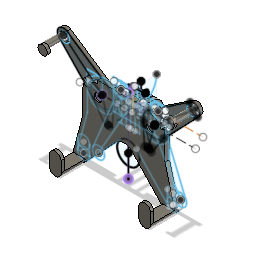
phone_holder (Autodesk Fusion 360 design; units mm, degrees)
Autodesk Fusion 360 part; units mm, degrees
sketch "Sketch1" plane through (0, 0, 0) normal (0, 0, 1) x (1, 0, 0)
  line L0 (-0.0193, 69.85) -> (19.0307, 69.85)
  line L1 (19.0307, 69.85) -> (19.0307, 50.8)
  line L2 (19.0307, 50.8) -> (-0.0193, 50.8)
  line L3 (-0.0193, 50.8) -> (-0.0193, 69.85)
  line L4 (3.7907, 69.85) -> (3.7907, 50.8)
  line L5 (7.6007, 69.85) -> (7.6007, 50.8)
  line L6 (11.4107, 69.85) -> (11.4107, 50.8)
  line L7 (15.2207, 69.85) -> (15.2207, 50.8)
  line L8 (-0.0193, 50.8) -> (-25.4193, 6.8059)
  line L9 (-0.0193, 50.8) -> (-41.2667, 50.8) construction
  line L10 (19.0307, 50.8) -> (44.4307, 6.8059)
  line L11 (19.0307, 50.8) -> (57.15, 50.8) construction
  circle A0 centre (-25.4193, 6.8059) radius 2.54
  circle A1 centre (44.4307, 6.8059) radius 2.54
  circle A2 centre (-25.4193, 6.8059) radius 5.08
  circle A3 centre (44.4307, 6.8059) radius 5.08
  line L12 (-12.7193, 68.9588) -> (31.7307, 68.9588)
  line L13 (31.7307, 68.9588) -> (31.7307, 43.5588)
  line L14 (31.7307, 43.5588) -> (-12.7193, 43.5588)
  line L15 (-12.7193, 43.5588) -> (-12.7193, 68.9588)
  line L16 (-12.7193, 50.8) -> (-30.1136, 8.7476)
  line L17 (31.7307, 50.8) -> (49.1249, 8.7476)
  circle A4 centre (-6.3693, 62.6088) radius 1.5875
  circle A5 centre (25.3807, 62.6088) radius 1.5875
  line L18 (-6.3693, 62.6088) -> (31.75, 62.6088) construction
  line L19 (25.3807, 62.6088) -> (63.5, 62.6088) construction
  circle A6 centre (-6.3693, 62.6088) radius 6.35
  circle A7 centre (25.3807, 62.6088) radius 6.35
  circle A8 centre (25.3807, 62.6088) radius 5.715
  circle A9 centre (-6.3693, 62.6088) radius 5.715
  line L20 (-6.3693, 68.9588) -> (-6.3693, 62.6088)
  line L21 (25.3807, 68.9588) -> (25.3807, 62.6088)
  line L22 (25.3807, 62.6088) -> (31.2629, 66.005)
  line L23 (25.3807, 62.6088) -> (31.75, 62.6088) construction
  line L24 (-6.3693, 62.6088) -> (-12.2226, 65.9882)
  line L25 (-6.3693, 62.6088) -> (-2.5108, 62.6088) construction
  circle A10 centre (25.3807, 62.6088) radius 1.4605
  circle A11 centre (-6.3693, 62.6088) radius 1.4605
  line L26 (29.6822, 66.3715) -> (31.731, 66.3715) construction
  line L27 (25.3807, 62.6088) -> (38.0807, 62.6088) construction
  line L28 (-6.3693, 62.6088) -> (12.6807, 62.6088) construction
  point P0 (-6.3693, 62.6088)
  point P1 (25.3807, 62.6088)
  dimension "d1" = 19.05
  dimension "d2" = 3.81
  dimension "d3" = 3.81
  dimension "d4" = 3.81
  dimension "d5" = 3.81
  dimension "d6" = 19.05
  dimension "d7" = 50.8
  dimension "d10" = 120
  dimension "d11" = 50.8
  dimension "d12" = 60
  dimension "d13" = 50.8
  dimension "d14" = 5.08
  dimension "d15" = 5.08
  dimension "d16" = 10.16
  dimension "d17" = 10.16
  dimension "d19" = 44.45
  dimension "d21" = 12.7
  dimension "d34" = 6.35
  dimension "d35" = 6.35
  dimension "d36" = 3.175
  dimension "d37" = 3.175
  dimension "d42" = 12.7
  dimension "d43" = 12.7
  dimension "d44" = 6.35
  dimension "d45" = 11.43
  dimension "d46" = 11.43
  dimension "d47" = 30
  dimension "d48" = 150
  dimension "d53" = 2.921
  dimension "d60" = 2.921
  constraint horizontal L0
  constraint vertical L1
  constraint horizontal L2
  constraint vertical L3
  constraint coincident L0 L4.start
  constraint coincident L2 L4.end
  constraint perpendicular L2 L4
  constraint coincident L0 L5.start
  constraint coincident L2 L5.end
  constraint perpendicular L2 L5
  constraint coincident L0 L6.start
  constraint coincident L2 L6.end
  constraint perpendicular L2 L6
  constraint coincident L0 L7.start
  constraint coincident L2 L7.end
  constraint perpendicular L2 L7
  constraint horizontal L9
  constraint horizontal L11
  constraint coincident L8.end A0.centre
  constraint coincident L10.end A1.centre
  constraint concentric A0 A2
  constraint concentric A1 A3
  constraint horizontal L12
  constraint vertical L13
  constraint horizontal L14
  constraint vertical L15
  constraint coincident L9 L16.start
  constraint coincident L15 L16.start
  constraint coincident A2 L16.end
  constraint tangent A2 L16
  constraint coincident L11 L17.start
  constraint coincident L13 L17.start
  constraint coincident A3 L17.end
  constraint tangent A3 L17
  constraint horizontal P0 P1
  constraint coincident P0 A4.centre
  constraint coincident P1 A5.centre
  constraint horizontal L18
  constraint horizontal L19
  constraint concentric A4 A6
  constraint concentric A5 A7
  constraint coincident L12 L20.start
  constraint coincident A6 L20.start
  constraint coincident L12 L21.start
  constraint coincident A7 L21.start
  constraint perpendicular L18 L21
  constraint horizontal L23
  constraint horizontal L25
  constraint concentric A7 A10
  constraint horizontal L26
  constraint coincident A8 L26.start
  constraint horizontal L27
  constraint horizontal L28
  measures "d1" distance of L0.start L2.end
  measures "d2" distance of L0.start L4
  measures "d3" distance of L4 L5
  measures "d4" distance of L5 L6
  measures "d5" distance of L6 L7
  measures "d6" distance of L1 L3
  measures "d7" distance of origin L2
  measures "d10" angle of L8 L9
  measures "d11" distance of L2.end L8.end
  measures "d12" angle of L10 L11
  measures "d13" distance of L1.end L10.end
  measures "d14" diameter of A0
  measures "d15" diameter of A1
  measures "d16" diameter of A2
  measures "d17" diameter of A3
  measures "d19" distance of L12.start L12.end
  measures "d21" horizontal distance of L0.start L12.start
  measures "d34" distance of L12 P0
  measures "d35" horizontal distance of L12.start P0
  measures "d36" diameter of A4
  measures "d37" diameter of A5
  measures "d42" diameter of A6
  measures "d43" diameter of A7
  measures "d44" distance of L13 P1
  measures "d45" diameter of A8
  measures "d46" diameter of A9
  measures "d47" angle of L22 L23
  measures "d48" angle of L24 L25
  measures "d53" diameter of A10
  measures "d60" diameter of A11
sketch "Sketch2" plane through (3.7907, 0, 0) normal (-1, 0, 0) x (0, 0, 1)
  line L0 (0, 68.9588) -> (-20.32, 68.9588)
  line L1 (-20.32, 68.9588) -> (-20.32, 50.8)
  line L2 (-20.32, 50.8) -> (0, 50.8)
  circle A0 centre (-10.795, 59.8794) radius 2.54
  arc A1 (-20.3135, 68.9588) -> (-2.7389, 50.8) centre (-1.6346, 69.4527) ccw
  line L3 (0, 50.8) -> (0, 68.9588)
  point P0 (-10.795, 59.8794)
  point P1 (0, 69.85)
  dimension "d125" = 9.525
  dimension "d126" = 5.08
  dimension "d127" = 9.0794
  constraint coincident P0 A0.centre
  constraint tangent L1 A1
  constraint coincident L2 A1.end
  constraint coincident L0 A1.start
  measures "d125" horizontal distance of L0.end P0
  measures "d126" diameter of A0
  measures "d127" distance of L0 P0
sketch "Sketch3" plane through (0, 0, 0) normal (0, 0, 1) x (1, 0, 0)
  line L0 (0, 0) -> (0, 63.5)
  line L1 (-9.525, 63.5092) -> (0, 63.5)
  circle A0 centre (0, 19.05) radius 9.525
  circle A1 centre (-38.0999, 0.0651) radius 2.54
  circle A2 centre (-38.0999, 0.0651) radius 5.08
  line L2 (-34.4118, -3.4284) -> (-6.9152, 25.6002)
  line L3 (-9.525, 63.5092) -> (-34.925, 63.5092)
  line L4 (-34.925, 63.5092) -> (-34.925, 31.7592)
  line L5 (-34.925, 31.7592) -> (-43.0092, 1.3711)
  line L6 (-9.525, 63.5092) -> (-9.525, 38.1092)
  line L7 (-9.525, 38.1092) -> (0, 38.1092)
  line L8 (-9.525, 57.1592) -> (0, 57.1592)
  line L9 (-5.715, 57.1592) -> (-5.715, 38.1092)
  line L10 (-1.905, 57.1592) -> (-1.905, 38.1092)
  circle A3 centre (-22.225, 50.8092) radius 12.7
  circle A4 centre (-22.225, 50.8092) radius 10.16
  line L11 (-22.225, 50.8092) -> (-22.225, 63.5092)
  line L12 (-22.225, 50.8092) -> (-34.1591, 55.1529)
  line L13 (-22.225, 50.8092) -> (-9.525, 50.8092) construction
  circle A5 centre (-22.225, 50.8092) radius 1.4605
  line L14 (9.525, 63.5092) -> (9.525, 38.1092)
  line L15 (34.925, 31.7592) -> (43.0092, 1.3711)
  line L16 (9.525, 63.5092) -> (34.925, 63.5092)
  circle A6 centre (38.0999, 0.0651) radius 2.54
  line L17 (9.525, 57.1592) -> (0, 57.1592)
  line L18 (34.4118, -3.4284) -> (6.9152, 25.6002)
  line L19 (5.715, 57.1592) -> (5.715, 38.1092)
  line L20 (22.225, 50.8092) -> (22.225, 63.5092)
  line L21 (1.905, 57.1592) -> (1.905, 38.1092)
  line L22 (22.225, 50.8092) -> (34.1591, 55.1529)
  circle A7 centre (22.225, 50.8092) radius 12.7
  circle A8 centre (0, 19.05) radius 9.525
  line L23 (9.525, 63.5092) -> (0, 63.5)
  circle A9 centre (22.225, 50.8092) radius 1.4605
  line L24 (34.925, 63.5092) -> (34.925, 31.7592)
  circle A10 centre (38.0999, 0.0651) radius 5.08
  line L25 (9.525, 38.1092) -> (0, 38.1092)
  circle A11 centre (22.225, 50.8092) radius 10.16
  line L26 (22.225, 50.8092) -> (9.525, 50.8092) construction
  circle A12 centre (-38.0999, 8.359) radius 5.08
  line L27 (-43.1364, 9.0231) -> (-43.1799, 0.0898)
  line L28 (-33.0635, 9.0231) -> (-33.02, 0.0898)
  circle A13 centre (38.0999, 8.359) radius 5.08
  line L29 (33.0635, 9.0231) -> (33.02, 0.0898)
  line L30 (43.1364, 9.0231) -> (43.1799, 0.0898)
  line L31 (43.1799, 0.0898) -> (33.02, 0.0898)
  line L32 (-33.02, 0.0898) -> (-43.1799, 0.0898)
  circle A14 centre (-22.225, 50.8092) radius 3.175
  circle A15 centre (22.225, 50.8092) radius 3.175
  point P0 (-38.0999, 0.0651)
  point P1 (13.8708, 60.4993)
  point P2 (-22.225, 50.8092)
  point P3 (22.225, 50.8092)
  point P4 (38.0999, 0.0651)
  dimension "d130" = 63.5
  dimension "d131" = 38.1
  dimension "d134" = 19.05
  dimension "d135" = 19.05
  dimension "d136" = 5.08
  dimension "d137" = 10.16
  dimension "d138" = 25.4
  dimension "d139" = 31.75
  dimension "d140" = 25.4
  dimension "d141" = 6.35
  dimension "d145" = 12.7
  dimension "d146" = 12.7
  dimension "d148" = 3.81
  dimension "d149" = 3.81
  dimension "d150" = 25.4
  dimension "d151" = 20.32
  dimension "d152" = 160
  dimension "d153" = 2.921
  dimension "d159" = 10.16
  dimension "d166" = 6.35
  constraint coincident L0.start origin
  constraint vertical L0
  constraint coincident L0 A0.centre
  constraint coincident P0 A1.centre
  constraint coincident A2 L2.start
  constraint coincident A0 L2.end
  constraint tangent A0 L2
  constraint tangent A2 L2
  constraint perpendicular L3 L4
  constraint coincident A2 L5.end
  constraint tangent A2 L5
  constraint perpendicular L3 L6
  constraint coincident L0 L7.end
  constraint perpendicular L0 L7
  constraint coincident L6 L8.start
  constraint coincident L0 L8.end
  constraint perpendicular L0 L8
  constraint coincident L8 L9.start
  constraint coincident L7 L9.end
  constraint perpendicular L7 L9
  constraint coincident L8 L10.start
  constraint coincident L7 L10.end
  constraint perpendicular L7 L10
  constraint coincident P2 A3.centre
  constraint midpoint L3 L11.end
  constraint horizontal L13
  constraint concentric A3 A5
  constraint symmetric L1.end L0 L23.end
  constraint symmetric L0 P0 P4
  constraint symmetric L0 L1.start L14.start
  constraint symmetric L0 A0 A8
  constraint symmetric L0 A1 A6
  constraint symmetric L0 A2 A10
  constraint symmetric L0 L2.start L18.start
  constraint symmetric L0 L2.end L18.end
  constraint symmetric L0 L3.end L16.end
  constraint symmetric L0 L4.end L15.start
  constraint symmetric L0 L5.end L15.end
  constraint symmetric L0 L6.end L14.end
  constraint symmetric L0 L7.end L25.end
  constraint symmetric L0 L8.start L17.start
  constraint symmetric L0 L8.end L17.end
  constraint symmetric L0 P2 P3
  constraint symmetric L0 L9.start L19.start
  constraint symmetric L0 L9.end L19.end
  constraint symmetric L0 L10.start L21.start
  constraint symmetric L0 L10.end L21.end
  constraint symmetric L0 A3 A7
  constraint symmetric L0 A4 A11
  constraint symmetric L0 L11.end L20.end
  constraint symmetric L0 L12.end L22.end
  constraint symmetric L0 L13.end L26.end
  constraint symmetric L0 A5 A9
  constraint coincident A12 L27.start
  constraint coincident A2 L27.end
  constraint tangent A2 L27
  constraint coincident A12 L28.start
  constraint coincident A2 L28.end
  constraint tangent A2 L28
  constraint symmetric L0 A12 A13
  constraint symmetric L0 L27.start L30.start
  constraint symmetric L0 L27.end L30.end
  constraint symmetric L0 L28.start L29.start
  constraint symmetric L0 L28.end L29.end
  constraint horizontal L31
  constraint symmetric L0 A14 A15
  measures "d130" distance of L0.start L0.end
  measures "d131" distance of L0.start P0
  measures "d134" diameter of A0
  measures "d135" distance of L0.start A0.centre
  measures "d136" diameter of A1
  measures "d137" diameter of A2
  measures "d138" distance of L1.start L3.end
  measures "d139" distance of L3.end L4.end
  measures "d140" distance of L1.start L6.end
  measures "d141" distance of L1.start L8.start
  measures "d145" distance of L4 P2
  measures "d146" distance of L3 P2
  measures "d148" distance of L6 L9
  measures "d149" distance of L9 L10
  measures "d150" diameter of A3
  measures "d151" diameter of A4
  measures "d152" angle of L12 L13
  measures "d153" diameter of A5
  measures "d159" diameter of A12
  measures "d166" diameter of A14
extrude "Extrude27" add sketch "Sketch3" along normal blind 3.81 contours L0 L7 L8 L10 | L0 A0 L14 L15 L18 A7 A8 L24 A10 L25 A13 L29 | L0 A0 A2 L2 L4 L5 L6 L7 A3 A8 A12 L28 | L0 L17 L21 L25 | L0 L1 L6 L8 | L0 L14 L17 L23 | L7 L8 L9 L10 | L17 L19 L21 L25 | L6 L7 L8 L9 | L14 L17 L19 L25 | L3 L6 A3 | L14 L16 A7 | A6 A10 L31 | A1 A2 L32 | A3 A4 L11 L12 | L20 L22 A7 A11 | A10 A13 L29 | A6 A10 A13 L31 | A1 A2 A12 L32 | A4 L11 L12 A14 | A4 L11 L12 A14 | L20 L22 A11 A15 | L20 L22 A11 A15 | L15 A10 A13 L29 | A10 A13 | A13 L29 | A6 L31 | A6 L31 | A2 L5 A12 | A1 L32 | A1 L32 | A2 A12 L28 | L11 L12 A5 A14 | L11 L12 A5 A14 | L20 L22 A9 A15 | L20 L22 A9 A15 | L15 A10 A13 | A2 L5 A12 L28 | A2 A12 | A12 L28 picked at (-32.4698, 44.8944) picked at (10.423, 50.0121) makes body 1
extrude "Extrude28" add sketch "Sketch3" against normal blind 20.32 contours L0 L7 L8 L10 | L0 L17 L21 L25 | L6 L7 L8 L9 | L14 L17 L19 L25 bodies 1
extrude "Extrude29" add sketch "Sketch3" along normal blind 21.59 contours A6 A10 L31 | A1 A2 L32 | A6 L31 | A1 L32 picked at (37.3916, -0.4969) picked at (-37.3149, -0.7364) bodies 1
extrude "Extrude30" add sketch "Sketch3" along normal blind 24.13 and the other way blind -21.59 contours A6 A10 L31 | A1 A2 L32 | A10 A13 L29 | A6 A10 A13 L31 | A2 L5 A12 L27 | A1 A2 A12 L32 | L15 A10 A13 L29 | A10 A13 | A13 L29 | A6 L31 | A6 L31 | L15 A10 A13 L30 | A2 L5 A12 | L5 A12 L27 | A12 L27 | A1 L32 | A1 L32 | A2 A12 L28 | L15 A10 A13 | L15 A13 L30 | A2 L5 A12 L28 | A2 A12 bodies 1
extrude "Extrude31" cut sketch "Sketch3" along normal blind 5.08 and the other way blind -2.54 contours L11 L12 A5 A14 | L11 L12 A5 A14 | L20 L22 A9 A15 | L20 L22 A9 A15 bodies 1
sketch "Sketch4" plane through (0, 0, 0) normal (0, 0, 1) x (1, 0, 0)
  line L0 (-9.525, 38.1092, -20.32) -> (-9.525, 57.1592, -20.32)
  circle A0 through (-9.525, 57.1592, -10.795) (-9.525, 42.8717, -2.5461) (-9.525, 42.8717, -19.0439)
  line L1 (-9.525, 57.1592, -20.32) -> (-9.525, 38.1092, -20.32)
  line L2 (-9.525, 38.1092, -20.32) -> (-9.525, 38.1092, 0)
  line L3 (-9.525, 38.1092) -> (-9.525, 57.1592)
  line L4 (-9.525, 57.1592, 0) -> (-9.525, 57.1592, -20.32)
  circle A1 through (-9.525, 50.1742, -10.795) (-9.525, 46.3642, -8.5953) (-9.525, 46.3642, -12.9947)
  point P0 (-9.525, 47.6342)
  dimension "d171" = 9.525
  dimension "d172" = 19.05
  dimension "d173" = 19.05
  dimension "d174" = 20.32
  dimension "d175" = 5.08
  constraint vertical L3
  measures "d173" distance of L3.end L3.start
extrude "Extrude32" cut sketch "Sketch4" along normal blind 19.05 contours L0 A0 L1 L2 | L0 A0 L1 L4 | A1 in plane through (-9.525, 0, 0) normal (1, 0, 0) bodies 1
sketch "Sketch5" plane through (0, 0, 0) normal (0, 0, 1) x (1, 0, 0)
  circle A0 centre (-22.225, 50.8092) radius 9.8425
  line L0 (-22.225, 50.8092) -> (3.175, 50.8092) construction
  line L1 (-22.225, 50.8092) -> (-16.9658, 31.1816)
  line L2 (-22.225, 50.8092) -> (-3.175, 50.8092) construction
  circle A1 centre (-16.9658, 31.1816) radius 1.27
  circle A2 centre (-16.9658, 31.1816) radius 3.175
  line L3 (-30.3699, 45.2833) -> (-19.5932, 29.3991)
  line L4 (-12.4084, 50.0961) -> (-13.7991, 30.9516)
  line L5 (-13.293, 46.6748) -> (-19.8471, 32.5153)
  circle A3 centre (-22.225, 50.8092) radius 0.9525
  circle A4 centre (-22.225, 50.8092) radius 2.8575
  line L6 (0, 0) -> (0, 63.5)
  circle A5 centre (22.225, 50.8092) radius 0.9525
  circle A6 centre (16.9658, 31.1816) radius 3.175
  line L7 (22.225, 50.8092) -> (3.175, 50.8092) construction
  circle A7 centre (16.9658, 31.1816) radius 1.27
  circle A8 centre (22.225, 50.8092) radius 2.8575
  line L8 (30.3699, 45.2833) -> (19.5932, 29.3991)
  line L9 (22.225, 50.8092) -> (16.9658, 31.1816)
  circle A9 centre (22.225, 50.8092) radius 9.8425
  line L10 (13.293, 46.6748) -> (19.8471, 32.5153)
  line L11 (12.4084, 50.0961) -> (13.7991, 30.9516)
  line L12 (-22.225, 50.8092) -> (-55.3028, 78.5648)
  line L13 (-22.225, 50.8092) -> (19.05, 50.8092) construction
  circle A10 centre (-55.3028, 78.5648) radius 2.54
  circle A11 centre (-55.3028, 78.5648) radius 5.08
  line L14 (-52.4866, 82.7927) -> (-16.7686, 59.0008)
  line L15 (-58.9774, 75.0572) -> (-29.3446, 44.0132)
  line L16 (-34.5322, 58.4836) -> (-22.225, 50.8092)
  line L17 (-30.5009, 57.7536) -> (-31.3018, 56.4692)
  line L18 (-34.5322, 58.4836) -> (-33.2261, 60.0402)
  arc A12 (-57.8401, 78.4483) -> (-55.6777, 81.077) centre (-53.9938, 77.4879) ccw
  circle A13 centre (22.225, 50.8092) radius 0.9525
  circle A14 centre (22.225, 50.8092) radius 2.8575
  line L19 (34.5322, 58.4836) -> (33.2261, 60.0402)
  line L20 (30.5009, 57.7536) -> (31.3018, 56.4692)
  line L21 (34.5322, 58.4836) -> (22.225, 50.8092)
  circle A15 centre (55.3028, 78.5648) radius 2.54
  circle A16 centre (55.3028, 78.5648) radius 5.08
  line L22 (52.4866, 82.7927) -> (16.7686, 59.0008)
  line L23 (22.225, 50.8092) -> (55.3028, 78.5648)
  arc A17 (55.6777, 81.077) -> (57.8401, 78.4483) centre (53.9938, 77.4879) ccw
  line L24 (12.4084, 50.0961) -> (13.7991, 30.9516)
  line L25 (22.225, 50.8092) -> (16.9658, 31.1816)
  circle A18 centre (16.9658, 31.1816) radius 3.175
  circle A19 centre (16.9658, 31.1816) radius 1.27
  line L26 (58.9774, 75.0572) -> (29.3446, 44.0132)
  line L27 (30.3699, 45.2833) -> (19.5932, 29.3991)
  line L28 (13.293, 46.6748) -> (19.8471, 32.5153)
  circle A20 centre (22.225, 50.8092) radius 9.8425
  point P0 (-22.225, 50.8092)
  point P1 (-22.225, 50.8092)
  point P2 (22.225, 50.8092)
  point P3 (22.225, 50.8092)
  point P4 (-22.225, 50.8092)
  point P5 (22.225, 50.8092)
  point P6 (22.225, 50.8092)
  point P7 (22.225, 50.8092)
  dimension "d178" = 19.685
  dimension "d183" = 75
  dimension "d184" = 20.32
  dimension "d185" = 2.54
  dimension "d186" = 6.35
  dimension "d193" = 1.905
  dimension "d194" = 5.715
  dimension "d215" = 140
  dimension "d216" = 43.18
  dimension "d217" = 5.08
  dimension "d218" = 10.16
  dimension "d220" = 2.032
  dimension "d221" = 14.3609
  constraint coincident P4 P0
  constraint coincident P4 P1
  constraint horizontal L0
  constraint coincident P1 P0
  constraint horizontal L2
  constraint coincident L1.end A1.centre
  constraint coincident A0 L3.start
  constraint coincident A2 L3.end
  constraint tangent A2 L3
  constraint tangent A0 L3
  constraint coincident A0 L4.start
  constraint coincident A2 L4.end
  constraint tangent A2 L4
  constraint tangent A0 L4
  constraint coincident A0 L5.start
  constraint coincident A2 L5.end
  constraint tangent A2 L5
  constraint tangent A0 L5
  constraint symmetric P4 L6 P7
  constraint symmetric A0 L6 A9
  constraint symmetric L1.end L6 A6.centre
  constraint symmetric L2.end L6 L0.end
  constraint symmetric A1 L6 A7
  constraint symmetric A2 L6 A6
  constraint symmetric L3.start L6 L8.start
  constraint symmetric L3.end L6 L8.end
  constraint symmetric L4.start L6 L11.start
  constraint symmetric L4.end L6 L11.end
  constraint symmetric L5.start L6 L10.start
  constraint symmetric L5.end L6 L10.end
  constraint symmetric A3 L6 A5
  constraint symmetric A4 L6 A8
  constraint horizontal L13
  constraint coincident L12.end A10.centre
  constraint coincident A11 L14.start
  constraint coincident A0 L14.end
  constraint tangent A0 L14
  constraint coincident A11 L15.start
  constraint coincident A0 L15.end
  constraint tangent A0 L15
  constraint coincident L12 L17.start
  constraint coincident L16 L17.end
  constraint perpendicular L16 L17
  constraint coincident L12 L18.end
  constraint perpendicular L12 L18
  constraint tangent A11 L15
  constraint tangent A11 L14
  constraint coincident A10 A12.end
  constraint coincident A10 A12.start
  constraint symmetric A0 L6 A20
  constraint symmetric P1 L6 P7
  constraint symmetric A1 L6 A19
  constraint symmetric A2 L6 A18
  constraint symmetric A3 L6 A13
  constraint symmetric A4 L6 A14
  constraint symmetric L6 L12.end A15.centre
  constraint symmetric L6 A10 A15
  constraint symmetric L6 A11 A16
  constraint symmetric L6 L14.start L22.start
  constraint symmetric L6 L14.end L22.end
  constraint symmetric L6 L15.start L26.start
  constraint symmetric L6 L15.end L26.end
  constraint symmetric L6 L16.start L19.start
  constraint symmetric L6 P4 P7
  constraint symmetric L6 L17.start L20.start
  constraint symmetric L6 L17.end L20.end
  constraint symmetric L6 L18.end L19.end
  constraint symmetric L6 A12.start A17.end
  constraint symmetric L6 A12.end A17.start
  constraint symmetric L6 A12 A17
  measures "d178" diameter of A0
  measures "d183" angle of L1 L2
  measures "d184" distance of P4 L1.end
  measures "d185" diameter of A1
  measures "d186" diameter of A2
  measures "d193" diameter of A3
  measures "d194" diameter of A4
  measures "d215" angle of L12 L13
  measures "d216" distance of P1 L12.end
  measures "d217" diameter of A10
  measures "d218" diameter of A11
  measures "d220" distance of L16.start L18.end
  measures "d221" distance of L18 P4
extrude "Extrude37" cut sketch "Sketch3" along normal blind 0.635 contours L11 L12 A5 A14 | L11 L12 A5 A14 | L20 L22 A9 A15 | L20 L22 A9 A15 bodies 1
extrude "Extrude40" add sketch "Sketch5" against normal blind 1.27 separate body contours A0 L1 A2 L4 L5 | A2 | L1 A2 L5 | A6 L9 L10 L25 A18 L28 | A6 L9 A9 L10 L11 L24 L25 A18 L28 A20 | A6 A18 makes body 2 at (-16.7336, 37.2127, -1.27) makes body 3 at (16.7336, 37.2127, 0)
extrude "Extrude42" add sketch "Sketch5" against normal blind 3.175 contours A0 L1 A4 L12 | A0 L12 A11 L14 A12 | A0 A4 L12 L16 | A0 L12 L16 L17 | A10 A11 A12 | A0 L1 L5 | A0 L1 A4 L16 | A0 L3 L12 A11 L15 L16 L18 A12 | A3 A4 L12 L16 | L1 A3 A4 L12 | L12 L16 L17 L18 | L12 A11 A12 | L12 A10 A11 A12 | A0 L1 A2 L3 L5 L15 | L1 A3 A4 L16 | L12 A10 A11 A12 | L12 A11 A12 | A10 | A1 | A5 A8 L9 A13 A14 L21 L25 | A5 A8 A13 A14 L21 L23 | A5 A8 L9 A13 A14 L23 L25 | A8 L9 A9 A14 L21 L25 A20 | A8 A9 A14 L21 L23 A20 | A8 L9 A9 A14 L23 L25 A20 | L8 A9 L19 L21 A16 L23 A17 L26 L27 A20 | A9 L20 L21 L23 A20 | A6 L8 L9 A9 L10 L25 A18 L26 L27 L28 A20 | L9 A9 L10 L25 L28 A20 | A9 A16 L22 L23 A17 A20 | L19 L20 L21 L23 | A15 A16 A17 | A15 A16 L23 A17 | A16 L23 A17 | A16 L23 A17 | A15 A16 L23 A17 | A15 | A7 A19 bodies 2 3
extrude "Extrude43" add sketch "Sketch5" along normal blind 16.51 contours A10 | A15 bodies 2 3
extrude "Extrude44" add sketch "Sketch5" along normal blind 19.05 and the other way blind -16.51 contours L12 A11 A12 | L12 A10 A11 A12 | L12 A10 A11 A12 | L12 A11 A12 | A10 | A15 A16 L23 A17 | A16 L23 A17 | A16 L23 A17 | A15 A16 L23 A17 | A15 bodies 2 3
extrude "Extrude45" add sketch "Sketch5" along normal blind 3.81 contours L12 L16 L17 L18 | L19 L20 L21 L23 bodies 2 3
extrude "Extrude46" add sketch "Sketch5" along normal blind 0.635 contours A3 A4 L12 L16 | L1 A3 A4 L12 | L1 A3 A4 L16 | A5 A8 L9 A13 A14 L21 L25 | A5 A8 A13 A14 L21 L23 | A5 A8 L9 A13 A14 L23 L25 bodies 2 3
named bodies: "main_bracket", "left_arm", "right_arm"
